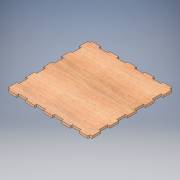
# Autodesk Inventor part: Bottom
Saved by Autodesk Inventor 2017.3 (Build 213256000, 256)
## iProperties
Created: 2019-04-26
Part Number: Bottom
Material: Wood (Birch)
Document SubType Name: Modeling
Designer: guberti
Density: 0.55 g/cm^3
Appearance: Birch - Natural Polished
Author: guberti
Autodesk Inventor part; units mm, degrees
ref_plane "YZ Plane" through (0, 0, 0) normal (1, 0, 0) x (0, 1, 0)
ref_plane "XZ Plane" through (0, 0, 0) normal (0, 1, 0) x (-1, 0, 0)
ref_plane "XY Plane" through (0, 0, 0) normal (0, 0, 1) x (1, 0, 0)
sketch "Sketch1" plane through (0, 0, 0) normal (0, 1, 0) x (-1, 0, 0)
  line L0 (0, 0) -> (-11.9062, 0)
  line L1 (-11.9062, 0) -> (-11.9062, -50.8)
  line L2 (-11.9062, -50.8) -> (0, -50.8)
  line L3 (0, -50.8) -> (0, -101.6)
  line L4 (0, -101.6) -> (-11.9062, -101.6)
  line L5 (-11.9062, -101.6) -> (-11.9062, -152.4)
  line L6 (-11.9062, -152.4) -> (0, -152.4)
  line L7 (0, -152.4) -> (0, -203.2)
  line L8 (0, -203.2) -> (-11.9062, -203.2)
  line L9 (0, 0) -> (0, 11.9062)
  line L10 (0, 11.9062) -> (50.8, 11.9062)
  line L11 (50.8, 11.9062) -> (50.8, 0)
  line L12 (50.8, 0) -> (101.6, 0)
  line L13 (101.6, 0) -> (101.6, 11.9062)
  line L14 (101.6, 11.9062) -> (152.4, 11.9062)
  line L15 (152.4, 11.9062) -> (152.4, 0)
  line L16 (152.4, 0) -> (203.2, 0)
  line L17 (203.2, 0) -> (203.2, 11.9062)
  line L18 (0, -457.2) -> (0, -469.1063)
  line L19 (50.8, -457.2) -> (101.6, -457.2)
  line L20 (50.8, -469.1063) -> (50.8, -457.2)
  line L21 (0, -469.1063) -> (50.8, -469.1063)
  line L22 (0, -457.2) -> (-11.9063, -457.2)
  line L23 (-11.9063, -457.2) -> (-11.9063, -406.4)
  line L24 (-11.9063, -406.4) -> (0, -406.4)
  line L25 (0, -406.4) -> (0, -355.6)
  line L26 (0, -355.6) -> (-11.9063, -355.6)
  line L27 (-11.9063, -355.6) -> (-11.9063, -304.8)
  line L28 (-11.9063, -304.8) -> (0, -304.8)
  line L29 (0, -304.8) -> (0, -254)
  line L30 (0, -254) -> (-11.9063, -254)
  line L31 (101.6, -457.2) -> (101.6, -469.1063)
  line L32 (101.6, -469.1063) -> (152.4, -469.1063)
  line L33 (152.4, -469.1063) -> (152.4, -457.2)
  line L34 (152.4, -457.2) -> (203.2, -457.2)
  line L35 (203.2, -457.2) -> (203.2, -469.1063)
  line L36 (457.2, -457.2) -> (469.1062, -457.2)
  line L37 (457.2, -406.4) -> (457.2, -355.6)
  line L38 (469.1062, -406.4) -> (457.2, -406.4)
  line L39 (469.1062, -457.2) -> (469.1062, -406.4)
  line L40 (457.2, -457.2) -> (457.2, -469.1062)
  line L41 (457.2, -469.1062) -> (406.4, -469.1062)
  line L42 (406.4, -469.1062) -> (406.4, -457.2)
  line L43 (406.4, -457.2) -> (355.6, -457.2)
  line L44 (355.6, -457.2) -> (355.6, -469.1062)
  line L45 (355.6, -469.1062) -> (304.8, -469.1062)
  line L46 (304.8, -469.1062) -> (304.8, -457.2)
  line L47 (304.8, -457.2) -> (254, -457.2)
  line L48 (254, -457.2) -> (254, -469.1062)
  line L49 (457.2, -355.6) -> (469.1062, -355.6)
  line L50 (469.1062, -355.6) -> (469.1062, -304.8)
  line L51 (469.1062, -304.8) -> (457.2, -304.8)
  line L52 (457.2, -304.8) -> (457.2, -254)
  line L53 (457.2, -254) -> (469.1062, -254)
  line L54 (457.2, 0) -> (457.2, 11.9063)
  line L55 (406.4, 0) -> (355.6, 0)
  line L56 (406.4, 11.9063) -> (406.4, 0)
  line L57 (457.2, 11.9063) -> (406.4, 11.9063)
  line L58 (457.2, 0) -> (469.1062, 0)
  line L59 (469.1062, 0) -> (469.1062, -50.8)
  line L60 (469.1062, -50.8) -> (457.2, -50.8)
  line L61 (457.2, -50.8) -> (457.2, -101.6)
  line L62 (457.2, -101.6) -> (469.1062, -101.6)
  line L63 (469.1062, -101.6) -> (469.1062, -152.4)
  line L64 (469.1062, -152.4) -> (457.2, -152.4)
  line L65 (457.2, -152.4) -> (457.2, -203.2)
  line L66 (457.2, -203.2) -> (469.1062, -203.2)
  line L67 (355.6, 0) -> (355.6, 11.9063)
  line L68 (355.6, 11.9063) -> (304.8, 11.9063)
  line L69 (304.8, 11.9063) -> (304.8, 0)
  line L70 (304.8, 0) -> (254, 0)
  line L71 (254, 0) -> (254, 11.9063)
  line L72 (254, 11.9063) -> (203.2, 11.9062)
  line L73 (-11.9062, -203.2) -> (-11.9063, -254)
  line L74 (203.2, -469.1063) -> (254, -469.1062)
  line L75 (469.1062, -203.2) -> (469.1062, -254)
  point P0 (228.6, -228.6)
  dimension "thickness" = 11.9062
  dimension "toothwidth" = 50.8
  dimension "d17" = 228.6
  dimension "d18" = 228.6
  dimension "d21" = 360
  constraints: 152 end point, 32 point on line, 13 perpendicular, 12 equal length, 3 horizontal, 1 parallel, 149 other
  measures "thickness" distance of L0.start L0.end
  measures "toothwidth" distance of L0.end L1.end
  measures "d17" horizontal distance of L0.start point (228.6, -228.6)
  measures "d18" horizontal distance of L0.start point (228.6, -228.6)
extrude "Extrusion1" add sketch "Sketch1" along normal blind 12.7
sketch "Sketch2" plane through (0, 0, 0) normal (0, -1, 0) x (1, 0, 0)
  line L0 (11.9062, -203.2) -> (11.9063, -254) construction
  line L1 (11.9063, -228.6) -> (-469.1062, -228.6) construction
  line L2 (-469.1062, -254) -> (-469.1062, -203.2) construction
  line L3 (-254, 11.9063) -> (-203.2, 11.9062) construction
  line L4 (-228.6, 11.9063) -> (-228.6, -469.1062) construction
  line L5 (-203.2, -469.1063) -> (-254, -469.1062) construction
  line L6 (0, 0) -> (-228.6, -228.6) construction
  line L7 (-25.4, -25.4) -> (-431.8, -25.4) construction
  line L8 (-431.8, -25.4) -> (-431.8, -431.8) construction
  line L9 (-431.8, -431.8) -> (-25.4, -431.8) construction
  line L10 (-25.4, -431.8) -> (-25.4, -25.4) construction
  line L11 (0, -254) -> (0, -304.8) construction
  line L12 (-152.4, -457.2) -> (-203.2, -457.2) construction
  line L13 (-212.1803, -194.2197) -> (-43.3605, -25.4)
  line L14 (-25.4, -43.3605) -> (-194.2197, -212.1803)
  arc A0 (-212.1803, -194.2197) -> (-228.6, -190.5) centre (-228.6, -228.6) ccw
  arc A1 (-190.5, -228.6) -> (-194.2197, -212.1803) centre (-228.6, -228.6) ccw
  line L15 (-245.0197, -194.2197) -> (-413.8395, -25.4)
  line L16 (-431.8, -43.3605) -> (-262.9803, -212.1803)
  arc A2 (-228.6, -190.5) -> (-245.0197, -194.2197) centre (-228.6, -228.6) ccw
  arc A3 (-262.9803, -212.1803) -> (-266.7, -228.6) centre (-228.6, -228.6) ccw
  line L17 (-212.1803, -262.9803) -> (-43.3605, -431.8)
  line L18 (-25.4, -413.8395) -> (-194.2197, -245.0197)
  arc A4 (-228.6, -266.7) -> (-212.1803, -262.9803) centre (-228.6, -228.6) ccw
  arc A5 (-194.2197, -245.0197) -> (-190.5, -228.6) centre (-228.6, -228.6) ccw
  line L19 (-431.8, -413.8395) -> (-262.9803, -245.0197)
  line L20 (-245.0197, -262.9803) -> (-413.8395, -431.8)
  arc A6 (-266.7, -228.6) -> (-262.9803, -245.0197) centre (-228.6, -228.6) ccw
  arc A7 (-245.0197, -262.9803) -> (-228.6, -266.7) centre (-228.6, -228.6) ccw
  line L21 (-43.3605, -25.4) -> (-413.8395, -25.4)
  line L22 (-431.8, -43.3605) -> (-431.8, -413.8395)
  line L23 (-413.8395, -431.8) -> (-43.3605, -431.8)
  line L24 (-25.4, -413.8395) -> (-25.4, -43.3605)
  dimension "border" = 25.4
  dimension "d27" = 25.4
  dimension "d28" = 38.1
  dimension "d29" = 38.1
  dimension "d30" = 12.7
  dimension "d31" = 12.7
  constraints: 38 end point, 16 point on circle, 14 symmetric about line, 8 centre point, 6 point on line, 5 midpoint, 3 collinear, 3 parallel, 2 perpendicular, 1 coincident, 1 horizontal, 6 other
  measures "border" distance between parallel lines of L10 L11
  measures "d27" distance between parallel lines of L12 L9
  measures "d28" radius of A1
  measures "d29" radius of A0
  measures "d30" distance between parallel lines of L13 L6
  measures "d31" distance between parallel lines of L14 L6
extrude "Extrusion2" cut sketch "Sketch2" against normal blind 9.525
fillet "Fillet1" radius 3.429 16 edges at (-194.2197, 4.7625, -245.0197) (-245.0197, 4.7625, -194.2197) (-413.8395, 4.7625, -25.4) (-43.3605, 4.7625, -25.4) (-25.4, 4.7625, -43.3605) (-25.4, 4.7625, -413.8395) (-43.3605, 4.7625, -431.8) (-431.8, 4.7625, -43.3605) (-262.9803, 4.7625, -212.1803) (-194.2197, 4.7625, -212.1803) (-212.1803, 4.7625, -194.2197) (-212.1803, 4.7625, -262.9803) (-245.0197, 4.7625, -262.9803) (-262.9803, 4.7625, -245.0197) (-431.8, 4.7625, -413.8395) (-413.8395, 4.7625, -431.8)
equation "\"d27\" = border"
equation "\"d30\" = 0.5 * border"
equation "\"d31\" = 0.5 * border"
body "Solid1"
